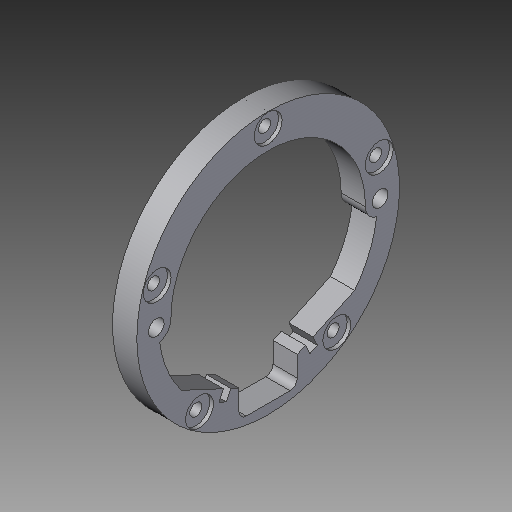
# Autodesk Inventor part: 3219_Center Rung_V1
Saved by Autodesk Inventor 2020 (Build 240168000, 168)
## iProperties
Created: 2018-08-02
Part Number: 3219_Center Rung_V1
Material: Acetal Resin, White
Document SubType Name: Modeling
Designer: em364
Density: 1.425 g/cm^3
Appearance: Smooth - White
Mass: 46.4909 g
Surface Area: 146.994 cm^2
Volume: 32.6252 cm^3
Author: em364
Autodesk Inventor part; units mm, degrees
ref_plane "YZ Plane" through (0, 0, 0) normal (1, 0, 0) x (0, 1, 0)
ref_plane "XZ Plane" through (0, 0, 0) normal (0, 1, 0) x (-1, 0, 0)
ref_plane "XY Plane" through (0, 0, 0) normal (0, 0, 1) x (1, 0, 0)
sketch "Sketch1" plane through (0, 0, 0) normal (1, 0, 0) x (0, 1, 0)
  circle A0 centre (-0.0138, -0.0327) radius 54
  circle A1 centre (-0.0138, 45.9673) radius 3.25
  circle A2 centre (-0.0138, -46.0327) radius 3.25
  arc A3 (-5.855, 44.5961) -> (-0.0138, 39.9673) centre (-0.0138, 45.9673) ccw
  arc A4 (-0.0138, -40.0327) -> (-5.8512, -44.6455) centre (-0.0138, -46.0327) ccw
  arc A5 (-0.0138, -40.0327) -> (-0.0138, 39.9673) centre (-0.0138, -0.0327) ccw
  line L0 (-38.5532, 11.9673) -> (-49.9975, 11.9673)
  line L1 (-49.9975, 11.9673) -> (-49.9975, -12.0327)
  line L2 (-38.5532, -12.0327) -> (-49.9975, -12.0327)
  arc A6 (-5.855, 44.5961) -> (-27.5449, 35.5747) centre (-0.0138, -0.0327) ccw
  arc A7 (-27.56, -35.6078) -> (-5.8512, -44.6455) centre (-0.0138, -0.0327) ccw
  line L3 (-36.9846, 15.3313) -> (-40.8817, 17.1485)
  line L4 (-40.8817, 17.1485) -> (-39.4448, 20.23)
  line L5 (-39.4448, 20.23) -> (-35.5477, 18.4127)
  line L6 (-35.5477, 18.4127) -> (-27.5449, 35.5747)
  line L7 (-36.9846, 15.3313) -> (-38.5532, 11.9673)
  line L8 (-36.9846, -15.3967) -> (-40.8817, -17.214)
  line L9 (-40.8817, -17.214) -> (-39.4448, -20.2954)
  line L10 (-39.4448, -20.2954) -> (-35.5477, -18.4782)
  line L11 (-36.9846, -15.3967) -> (-38.5532, -12.0327)
  line L12 (-35.5477, -18.4782) -> (-27.56, -35.6078)
  line L13 (-0.0138, -0.0327) -> (-40.1632, 18.6893)
  line L14 (-0.0138, -0.0327) -> (-40.1632, -18.7547)
  line L15 (-0.0138, -0.0327) -> (-50.798, -0.0327) construction
  line L16 (-0.0138, -0.0327) -> (50.7703, -0.0327) construction
  dimension "d4" = 6.5
  dimension "d5" = 6.5
  dimension "d25" = 24
  dimension "d27" = 4.3
  dimension "d28" = 3.4
  dimension "d31" = 4.3
  dimension "d32" = 3.4
  dimension "d39" = 90
  dimension "d40" = 90
  dimension "d41" = 90
  dimension "d42" = 90
  dimension "d44" = 90
  dimension "d45" = 90
  dimension "d67" = 40
  dimension "d68" = 40
  dimension "d70" = 4.3
  dimension "d71" = 1.7
  dimension "d72" = 4.3
  dimension "d73" = 90
  dimension "d74" = 90
  dimension "d76" = 108
  dimension "d81" = 40
  dimension "d93" = 46
  dimension "d94" = 46
  dimension "d95" = 6
  dimension "d96" = 6
  dimension "d97" = 180
  dimension "d98" = 12
  dimension "d99" = 12
  dimension "d100" = 25
  dimension "d101" = 25
  dimension "d102" = 1.7
  constraints: 34 end point, 10 point on circle, 9 perpendicular, 8 centre point, 5 concentric, 3 collinear, 2 midpoint, 1 coincident, 1 horizontal
  measures "d4" diameter of A2
  measures "d5" diameter of A1
  measures "d25" distance of L0.end L1.end
  measures "d27" distance of L4.end L5.end
  measures "d28" distance of L3.end L4.end
  measures "d31" distance of L8.start L8.end
  measures "d32" distance of L8.end L9.end
  measures "d39" angle of L5 L6
  measures "d40" angle of L4 L5
  measures "d41" angle of L3 L4
  measures "d42" angle of L3 L7
  measures "d44" angle of L9 L8
  measures "d45" angle of L9 L10
  measures "d67" distance from line of A0.centre L6
  measures "d68" distance from line of L12 A0.centre
  measures "d70" distance of L3.start L3.end
  measures "d71" distance between parallel lines of L5 L13
  measures "d72" distance of L9.end L10.end
  measures "d73" angle of L8 L11
  measures "d74" angle of L12 L10
  measures "d76" diameter of A0
  measures "d81" radius of A5
  measures "d93" distance of A2.centre A0.centre
  measures "d94" distance of A0.centre A1.centre
  measures "d95" radius of A3
  measures "d96" radius of A4
  measures "d97" angle of L15 L16
  measures "d98" distance from line of A0.centre L2
  measures "d99" distance from line of A6.centre L0
  measures "d100" angle of L15 L13
  measures "d101" angle of L14 L15
  measures "d102" distance between parallel lines of L8 L14
extrude "Extrusion1" add sketch "Sketch1" along normal blind 10
fillet "Fillet1" radius 3 2 edges at (5, -49.9975, 11.9673) (5, -49.9975, -12.0327)
sketch "Sketch2" plane through (10, -0.0138, -0.0327) normal (1, 0, 0) x (0, 0, -1)
  circle A0 centre (0, 0) radius 48
  circle A1 centre (0, 48) radius 2.5
  arc A2 (40, 0) -> (-40, 0) centre (0, 0) ccw projected
  arc A3 (40, 0) -> (44.6128, -5.8374) centre (46, 0) ccw projected
  arc A4 (35.575, -27.5462) -> (44.6128, -5.8374) centre (0, 0) ccw projected
  line L0 (35.575, -27.5462) -> (18.4455, -35.5339) projected
  line L1 (18.4455, -35.5339) -> (20.2627, -39.431) projected
  line L2 (20.2627, -39.431) -> (17.1813, -40.8679) projected
  line L3 (17.1813, -40.8679) -> (15.364, -36.9708) projected
  line L4 (15.364, -36.9708) -> (12, -38.5394) projected
  line L5 (12, -38.5394) -> (12, -46.9837) projected
  arc A5 (9, -49.9837) -> (12, -46.9837) centre (9, -46.9837) ccw projected
  line L6 (9, -49.9837) -> (-9, -49.9837) projected
  arc A6 (-12, -46.9837) -> (-9, -49.9837) centre (-9, -46.9837) ccw projected
  line L7 (-12, -46.9837) -> (-12, -38.5394) projected
  line L8 (-12, -38.5394) -> (-15.364, -36.9708) projected
  line L9 (-15.364, -36.9708) -> (-17.1813, -40.8679) projected
  line L10 (-17.1813, -40.8679) -> (-20.2627, -39.431) projected
  line L11 (-20.2627, -39.431) -> (-18.4455, -35.5339) projected
  line L12 (-18.4455, -35.5339) -> (-35.6074, -27.5311) projected
  arc A7 (-44.6288, -5.8412) -> (-35.6074, -27.5311) centre (0, 0) ccw projected
  arc A8 (-44.6288, -5.8412) -> (-40, 0) centre (-46, 0) ccw projected
  circle A9 centre (46, 0) radius 3.25 projected
  circle A10 centre (-46, 0) radius 3.25 projected
  circle A11 centre (0, 0) radius 54 projected
  circle A12 centre (0, 0) radius 54 projected
  circle A13 centre (-45.6507, 14.8328) radius 2.5
  circle A14 centre (-28.2137, -38.8328) radius 2.5
  circle A15 centre (28.2137, -38.8328) radius 2.5
  circle A16 centre (45.6507, 14.8328) radius 2.5
  point P0 (-0.0327, 0.0138)
  dimension "d50" = 96
  dimension "d51" = 5
  dimension "d80" = 108
  dimension "d84" = 360
  dimension "d103" = 0
  constraints: 5 centre point, 1 vertical alignment, 16 other
  measures "d51" diameter of A1
  measures "d80" diameter of A11
  measures "d103" horizontal distance of A11.centre A1.centre
extrude "Extrusion2" cut sketch "Sketch2" against normal blind 10 contours A16 A0 | A0 A16 | A15 A0 | A0 A15 | A1 A0 | A0 A1 | A13 A0 | A0 A13 | A14 A0 | A0 A14
sketch "Sketch3" plane through (10, -0.0138, -0.0327) normal (1, 0, 0) x (0, 0, -1)
  circle A0 centre (0, 48) radius 2.5 projected
  circle A1 centre (0, 48) radius 5.75
  circle A2 centre (0, 0) radius 54 projected
  circle A3 centre (-45.6507, 14.8328) radius 5.75
  circle A4 centre (-28.2137, -38.8328) radius 5.75
  circle A5 centre (28.2137, -38.8328) radius 5.75
  circle A6 centre (45.6507, 14.8328) radius 5.75
  point P0 (-0.0327, 0.0138)
  dimension "d58" = 11.5
  dimension "d88" = 360
  constraints: 5 centre point, 1 coincident, 11 other
  measures "d58" diameter of A1
extrude "Extrusion3" cut sketch "Sketch3" against normal blind 1.5 contours A1 | A3 | A4 | A5 | A6
sketch "Sketch6" plane through (0, -0.0138, -0.0327) normal (-1, 0, 0) x (0, 0, 1)
  circle A0 centre (0, 48) radius 5.75 projected
  circle A1 centre (-45.6507, 14.8328) radius 5.75 projected
  circle A2 centre (-28.2137, -38.8328) radius 5.75 projected
  circle A3 centre (28.2137, -38.8328) radius 5.75 projected
  circle A4 centre (45.6507, 14.8328) radius 5.75 projected
  point P0 (0.0327, 0.0138)
extrude "Extrusion5" cut sketch "Sketch6" against normal blind 1.5
equation "\"d98\" = 0.5 * d25"
body "Solid1"
